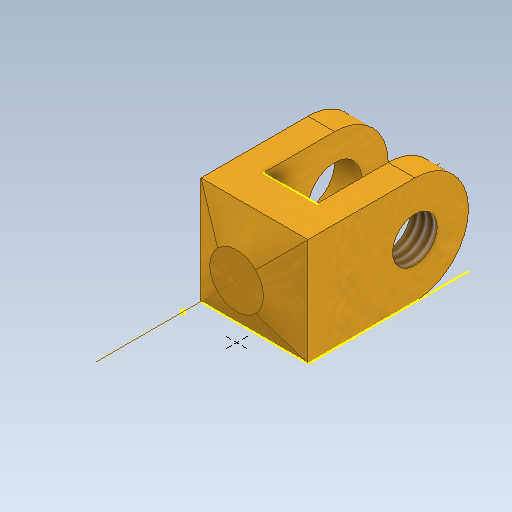
# Autodesk Inventor part: Part24
Saved by Autodesk Inventor 2020 (Build 240168000, 168)
## iProperties
Created: 2021-10-20
Part Number: Part24
Material: Brass, Soft Yellow, Welded
Document SubType Name: Modeling
Designer: simon.erikssonwestl
Density: 8.5 g/cm^3
Appearance: Weld - Brass
Author: simon.erikssonwestl
Autodesk Inventor part; units mm, degrees
ref_plane "YZ Plane" through (0, 0, 0) normal (1, 0, 0) x (0, 1, 0)
ref_plane "XZ Plane" through (0, 0, 0) normal (0, 1, 0) x (-1, 0, 0)
sketch "Sketch1" plane through (0, 0, 0) normal (0, 1, 0) x (-1, 0, 0)
  line L0 (0, 0) -> (-6, 0)
  line L1 (-6, 0) -> (-6, -9)
  line L2 (-6, -9) -> (0, -9)
  line L3 (0, -9) -> (0, 0)
  dimension "d0" = 6
  dimension "d1" = 9
  constraints: 8 end point, 2 parallel, 1 horizontal, 1 perpendicular
  measures "d0" distance of L2.end L1.end
  measures "d1" distance of L1.end L0.end
extrude "Extrusion1" add sketch "Sketch1" along normal blind 6
sketch "Sketch2" plane through (6, 0, -9) normal (0, 0, -1) x (-1, 0, 0)
  line L0 (0, 6) -> (6, 6) projected
  line L1 (0, 0) -> (6, 0) projected
  line L2 (1.5, 6) -> (4.5, 6)
  line L3 (4.5, 6) -> (4.5, 0)
  line L4 (4.5, 0) -> (1.5, 0)
  line L5 (1.5, 0) -> (1.5, 6)
  line L6 (0, 0) -> (0, 6) projected
  dimension "d4" = 3
  dimension "d5" = 1.5
  constraints: 8 end point, 2 parallel, 2 point on line, 1 horizontal, 1 perpendicular
  measures "d4" distance of L3.end L4.end
  measures "d5" distance between parallel lines of L6 L5
sketch "Sketch3" plane through (0, 0, 0) normal (0, -1, 0) x (1, 0, 0)
  line L0 (6, 0) -> (6, -9) projected
  line L1 (0, 0) -> (6, 0) projected
  point P0 (3, 1)
  dimension "d6" = 3
  dimension "d7" = 1
  measures "d6" distance from line of L0 point (3, 1)
  measures "d7" distance from line of L1 point (3, 1)
ref_plane "Work Plane1" through (3, 0, 1) normal (0, 0, 1) x (1, 0, 0)
sketch "Sketch4" plane through (3, 0, 1) normal (0, 0, 1) x (1, 0, 0)
  point P0 (-3, 0)
sketch "Sketch5" plane through (3, 0, 1) normal (0, 0, 1) x (1, 0, 0)
  circle A0 centre (0, 3) radius 1.5
  point P0 (-3, 0)
  dimension "d8" = 3
  constraints: 1 centre point
  measures "d8" diameter of A0
loft "Loft1" add profiles "Sketch5" section 1 edges at (3, 0, 0) (6, 3, 0) (3, 6, 0) (0, 3, 0)
extrude "Extrusion2" cut sketch "Sketch2" against normal blind 7 contours L0 L3 L1 L5
sketch "Sketch6" plane through (6, 0, -9) normal (1, 0, 0) x (0, 0, -1)
  line L0 (-9, 0) -> (-9, 6) projected
  line L1 (-9, 6) -> (0, 6) projected
  point P0 (-3, 3)
  dimension "d15" = 6
  dimension "d16" = 3
  measures "d15" distance from line of L0 point (-3, 3)
  measures "d16" distance from line of L1 point (-3, 3)
hole "Hole1" at (6, 3, -6) direction (-1, 0, 0) diameter 2.5 depth 1.5 tip angle 118
sketch "Sketch7" plane through (0, 0, -9) normal (-1, 0, 0) x (0, 0, 1)
  circle A0 centre (3, 3) radius 1.25 projected
  point P0 (9, 0)
  constraints: 1 coincident
hole "Hole2" at (0, 3, -6) at (0, 3, -6) direction (1, 0, 0) diameter 3 depth 1.5 tip angle 118
thread "Thread1" size "M2.5x0.45" class "6H" standard "ANSI Metric M Profile" full length
fillet "Fillet1" radius 3 4 edges at (5.25, 6, -9) (5.25, 0, -9) (0.75, 0, -9) (0.75, 6, -9)
sketch "Sketch8" plane through (6, 0, -2) normal (0, 0, -1) x (-1, 0, 0)
  line L0 (4.5, 6) -> (4.5, 0) projected
  line L1 (1.5, 6) -> (4.5, 6) projected
  line L2 (1.5, 0) -> (1.5, 6) projected
  line L3 (4.5, 0) -> (1.5, 0) projected
  point P0 (6, 0)
  point P1 (3, 3)
body "Solid1"
